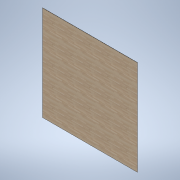
# Autodesk Inventor part: Piso
Saved by Autodesk Inventor 2020.3 (Build 243373000, 373)
## iProperties
Created: 2020-07-08
Part Number: Piso
Material: Wood (Maple)
Document SubType Name: Modeling
Designer: Bruno
Density: 0.67 g/cm^3
Appearance: Natural Maple - Glossy Dark Tint
Author: Bruno
Autodesk Inventor part; units mm, degrees
ref_plane "YZ Plane" through (0, 0, 0) normal (1, 0, 0) x (0, 1, 0)
ref_plane "XZ Plane" through (0, 0, 0) normal (0, 1, 0) x (-1, 0, 0)
ref_plane "XY Plane" through (0, 0, 0) normal (0, 0, 1) x (1, 0, 0)
sketch "Sketch1" plane through (0, 0, 0) normal (0, 0, 1) x (1, 0, 0)
  line L0 (2500, 2500) -> (-2500, 2500)
  line L1 (-2500, 2500) -> (-2500, -2500)
  line L2 (-2500, -2500) -> (2500, -2500)
  line L3 (2500, -2500) -> (2500, 2500)
  point P0 (0, 0)
  dimension "d0" = 5000
  dimension "d1" = 5000
  dimension "d2" = 2500
  dimension "d3" = 2500
  constraints: 8 end point, 2 parallel, 1 horizontal, 1 perpendicular
  measures "d0" distance of L0.start L0.end
  measures "d1" distance of L2.end L0.start
  measures "d2" distance from line of point (0, 0) L3
  measures "d3" distance from line of point (0, 0) L0
extrude "Extrusion1" add sketch "Sketch1" against normal blind 10
equation "\"d2\" = 0.5 * d1"
equation "\"d3\" = 0.5 * d0"
body "Solid1"
